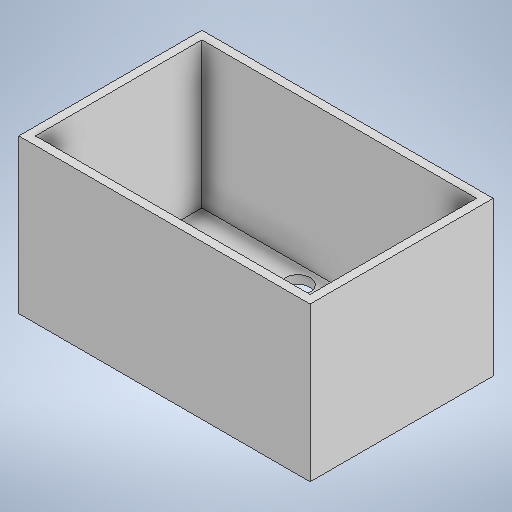
# Autodesk Inventor part: finalturnmotorcasing
Saved by Autodesk Inventor 2025.2 (Build 292293000, 293)
## iProperties
Created: 2026-03-25
Part Number: finalturnmotorcasing
Material: Generic
Document SubType Name: Modeling
Designer: hp
Density: 1 g/cm^3
Appearance: Default
Author: hp
Autodesk Inventor part; units mm, degrees
ref_plane "YZ Plane" through (0, 0, 0) normal (1, 0, 0) x (0, 1, 0)
ref_plane "XZ Plane" through (0, 0, 0) normal (0, 1, 0) x (-1, 0, 0)
ref_plane "XY Plane" through (0, 0, 0) normal (0, 0, 1) x (1, 0, 0)
sketch "Sketch1" plane through (0, 0, 0) normal (0, 1, 0) x (-1, 0, 0)
  line L0 (20.3745, 9.2758) -> (20.3745, -9.6242)
  line L1 (20.3745, 9.2758) -> (20.3745, -9.6242)
  circle A0 centre (24.4745, 4.8258) radius 2.25
  circle A1 centre (24.4745, 4.8258) radius 2.25
  line L2 (20.3745, 9.2758) -> (27.6745, 9.2758)
  line L3 (27.6745, 9.2758) -> (20.3745, 9.2758)
  line L4 (27.6745, 9.2758) -> (27.6745, -9.6242)
  line L5 (27.6745, 9.2758) -> (27.6745, -9.6242)
  circle A2 centre (24.4745, -5.1742) radius 2.25
  line L6 (20.3745, -9.6242) -> (27.6745, -9.6242)
  line L7 (27.6745, -9.6242) -> (20.3745, -9.6242)
  circle A3 centre (24.4745, -5.1742) radius 2.25
  line L8 (20.3745, 9.2758) -> (-20.1755, 9.2758)
  line L9 (20.3745, -9.6242) -> (-20.1755, -9.6242)
  line L10 (20.3745, 9.2758) -> (20.3745, -9.6242)
  line L11 (20.3745, 9.2758) -> (20.3745, -9.6242)
  line L12 (20.3745, 9.2758) -> (20.3745, -9.6242)
  line L13 (-20.1755, -9.6242) -> (20.3745, -9.6242)
  line L14 (-20.1755, -9.6242) -> (20.3745, -9.6242)
  line L15 (20.3745, 9.2758) -> (20.3745, -9.6242)
  line L16 (-20.1755, 9.2758) -> (20.3745, 9.2758)
  line L17 (-20.1755, 9.2758) -> (-20.1755, -9.6242)
  circle A4 centre (-10.3455, 0.2258) radius 6.5
  line L18 (20.3745, -9.6242) -> (-20.1755, -9.6242)
  line L19 (-20.1755, 9.2758) -> (-20.1755, -9.6242)
  line L20 (20.3745, 9.2758) -> (-20.1755, 9.2758)
  line L21 (20.3745, 9.2758) -> (20.3745, -9.6242)
  line L22 (20.3745, -9.6242) -> (-20.1755, -9.6242)
  line L23 (27.6745, -9.6242) -> (20.3745, -9.6242)
  line L24 (20.3745, -9.6242) -> (27.6745, -9.6242)
  line L25 (-20.1755, -9.6242) -> (20.3745, -9.6242)
  line L26 (-27.4755, -9.6242) -> (-20.1755, -9.6242)
  line L27 (-20.1755, -9.6242) -> (-27.4755, -9.6242)
  line L28 (-20.1755, 9.2758) -> (-27.4755, 9.2758)
  line L29 (-27.4755, 9.2758) -> (-20.1755, 9.2758)
  line L30 (-20.1755, 9.2758) -> (20.3745, 9.2758)
  line L31 (20.3745, 9.2758) -> (27.6745, 9.2758)
  line L32 (27.6745, 9.2758) -> (20.3745, 9.2758)
  line L33 (20.3745, 9.2758) -> (-20.1755, 9.2758)
  line L34 (-20.1755, 9.2758) -> (-20.1755, -9.6242)
  line L35 (-20.1755, 9.2758) -> (-20.1755, -9.6242)
  line L36 (-20.1755, 9.2758) -> (-20.1755, -9.6242)
  line L37 (-20.1755, 9.2758) -> (-20.1755, -9.6242)
  line L38 (-20.1755, 9.2758) -> (-20.1755, -9.6242)
  line L39 (-20.1755, 9.2758) -> (-20.1755, -9.6242)
  circle A5 centre (-24.3255, 4.8258) radius 2.25
  circle A6 centre (-24.3255, 4.8258) radius 2.25
  circle A7 centre (-24.3255, 4.8258) radius 2.25
  line L40 (-27.4755, 9.2758) -> (-20.1755, 9.2758)
  line L41 (-20.1755, -9.6242) -> (-27.4755, -9.6242)
  line L42 (-27.4755, 9.2758) -> (-27.4755, -9.6242)
  line L43 (-20.1755, 9.2758) -> (-27.4755, 9.2758)
  line L44 (-20.1755, 9.2758) -> (-20.1755, -9.6242)
  circle A8 centre (-24.3255, 4.8258) radius 2.25
  circle A9 centre (-24.3255, -5.1742) radius 2.25
  line L45 (-27.4755, -9.6242) -> (-20.1755, -9.6242)
  line L46 (-20.1755, 9.2758) -> (-20.1755, -9.6242)
  line L47 (-27.4755, 9.2758) -> (-20.1755, 9.2758)
  line L48 (-27.4755, 9.2758) -> (-27.4755, -9.6242)
  circle A10 centre (-24.3255, 4.8258) radius 2.25
  circle A11 centre (-24.3255, -5.1742) radius 2.25
  line L49 (-20.1755, 9.2758) -> (-20.1755, -9.6242)
  line L50 (-20.1755, 9.2758) -> (20.3745, 9.2758)
  circle A12 centre (-10.3455, 0.2258) radius 1.2002
  circle A13 centre (-10.3455, 0.2258) radius 2.9
  circle A14 centre (-10.3455, 0.2258) radius 6.5
  circle A15 centre (-10.3455, 0.2258) radius 6.5
  circle A16 centre (-10.3455, 0.2258) radius 6.5
  circle A17 centre (-10.3455, 0.2258) radius 6.5
  circle A18 centre (-10.3455, 0.2258) radius 2.9
  circle A19 centre (-10.3455, 0.2258) radius 6.5
  line L51 (-27.4755, 9.2758) -> (-27.4755, -9.6242)
  line L52 (-27.4755, 9.2758) -> (-27.4755, -9.6242)
  line L53 (-27.4755, 9.2758) -> (-27.4755, -9.6242)
  line L54 (-27.4755, 9.2758) -> (-27.4755, -9.6242)
  circle A20 centre (-24.3255, -5.1742) radius 2.25
  circle A21 centre (-24.3255, -5.1742) radius 2.25
  circle A22 centre (-24.3255, -5.1742) radius 2.25
  line L55 (-27.4755, -9.6242) -> (-20.1755, -9.6242)
  line L56 (-20.1755, -9.6242) -> (-27.4755, -9.6242)
  line L57 (20.3745, 9.2758) -> (20.3745, -9.6242)
  line L58 (20.3745, 9.2758) -> (20.3745, -9.6242)
  line L59 (20.3745, 9.2758) -> (20.3745, -9.6242)
  circle A23 centre (24.4745, 4.8258) radius 2.25
  circle A24 centre (24.4745, 4.8258) radius 2.25
  circle A25 centre (24.4745, -5.1742) radius 2.25
  circle A26 centre (24.4745, -5.1742) radius 2.25
  line L60 (27.6745, -9.6242) -> (20.3745, -9.6242)
  line L61 (20.3745, 9.2758) -> (20.3745, -9.6242)
  line L62 (27.6745, 9.2758) -> (20.3745, 9.2758)
  line L63 (27.6745, 9.2758) -> (27.6745, -9.6242)
  circle A27 centre (24.4745, 4.8258) radius 2.25
  circle A28 centre (24.4745, -5.1742) radius 2.25
  line L64 (20.3745, -9.6242) -> (27.6745, -9.6242)
  line L65 (27.6745, 9.2758) -> (27.6745, -9.6242)
  line L66 (20.3745, 9.2758) -> (27.6745, 9.2758)
  line L67 (20.3745, 9.2758) -> (20.3745, -9.6242)
  circle A29 centre (24.4745, 4.8258) radius 2.25
  circle A30 centre (24.4745, -5.1742) radius 2.25
  line L68 (27.6745, 9.2758) -> (27.6745, -9.6242)
  line L69 (27.6745, 9.2758) -> (27.6745, -9.6242)
  line L70 (-20.1755, 9.2758) -> (-20.1755, -9.6242)
  circle A31 centre (-10.3455, 0.2258) radius 1.2002
  circle A32 centre (-10.3455, 0.2258) radius 2.9
  circle A33 centre (-10.3455, 0.2258) radius 1.2002
  circle A34 centre (-10.3455, 0.2258) radius 2.9
  circle A35 centre (-10.3455, 0.2258) radius 1.2002
  circle A36 centre (-10.3455, 0.2258) radius 2.9
  circle A37 centre (-10.3455, 0.2258) radius 2.9
  circle A38 centre (-10.3455, 0.2258) radius 1.2002
  circle A39 centre (-10.3455, 0.2258) radius 1.2002
  circle A40 centre (-24.3255, 4.8258) radius 2.25
  circle A41 centre (-24.3255, -5.1742) radius 2.25
  line L71 (-20.1755, 9.2758) -> (-27.4755, 9.2758)
  line L72 (27.6745, -0.1742) -> (-27.4755, -0.1742)
  line L73 (0.0995, 9.2758) -> (0.0995, -9.6242)
  circle A42 centre (-10.3455, 0.2258) radius 20
  circle A43 centre (-10.3455, 0.2258) radius 22.5
  line L74 (-10.3455, 0.2258) -> (5.5644, -15.6841)
  line L75 (-10.3455, 0.2258) -> (12.1545, 0.2258) construction
  circle A44 centre (5.5644, -15.6841) radius 3
  circle A45 centre (5.5644, 16.1358) radius 3
  circle A46 centre (-26.2554, 16.1358) radius 3
  circle A47 centre (-26.2554, -15.6841) radius 3
  line L76 (35.0995, 21.8258) -> (-34.9005, 21.8258)
  line L77 (-34.9005, 21.8258) -> (-34.9005, -22.1742)
  line L78 (-34.9005, -22.1742) -> (35.0995, -22.1742)
  line L79 (35.0995, -22.1742) -> (35.0995, 21.8258)
  line L80 (35.0995, 21.8258) -> (-34.9005, -22.1742) construction
  line L81 (-34.9005, 21.8258) -> (35.0995, -22.1742) construction
  line L82 (33.0995, -20.1742) -> (-32.9005, -20.1742)
  line L83 (-32.9005, -20.1742) -> (-32.9005, 19.8258)
  line L84 (-32.9005, 19.8258) -> (33.0995, 19.8258)
  line L85 (33.0995, 19.8258) -> (33.0995, -20.1742)
  point P0 (0, 0)
  point P1 (0.0995, -0.1742)
  point P2 (-6.3655, 19.8258)
  point P3 (-14.3254, 19.8258)
  point P4 (-20.1755, -9.6242)
  dimension "d1" = 45
  dimension "d0" = 40
  dimension "d2" = 45
  dimension "d3" = 6
  dimension "d6" = 360
  dimension "d8" = 70
  dimension "d9" = 44
  dimension "d10" = 2
  constraints: 150 end point, 47 centre point, 7 midpoint, 4 parallel, 3 coincident, 2 horizontal, 2 perpendicular, 1 equal length, 48 other
  measures "d0" diameter of A42
  measures "d2" angle of L74 L75
  measures "d3" diameter of A44
  measures "d8" distance of L78.end L77.end
  measures "d9" distance of L77.end L76.end
  measures "d10" distance between parallel lines of L78 L82
extrude "Extrusion1" add sketch "Sketch1" against normal blind 2 contours L2 L4 L72 L0 | L8 A43 A45 L84 L85 L82 A44 L9 L6 L4 L2 | L0 L72 A43 L8 | L72 L4 L6 L0 | L0 L9 A43 L72 | A43 L72 A42 L8 | L8 A42 A45 A43 | A43 L9 A42 L72 | A42 L72 L73 L8 | L8 L28 L42 L26 L9 L74 A44 A42 A47 A46 L84 A45 | A43 A44 A42 L9 | A42 L9 L73 L72 | A45 A42 L84 A43 | A42 A44 L74 L9 | L17 L72 L42 L28 | L84 A42 A43 L76 | A43 L76 L79 L78 L82 L85 L84 | L17 L26 L42 L72 | L84 A42 | A43 L82 A47 A42 A44 | A42 A46 A43 L84 | A43 L84 L83 L82 L78 L77 L76 | A43 L78 L82 | A43 A46 A47 L82 L83 L84 | A42 A47 A43 A46
extrude "Extrusion2" add sketch "Sketch1" along normal blind 35 contours L84 A42 A43 L76 | A43 L76 L79 L78 L82 L85 L84 | L84 A42 | A43 L84 L83 L82 L78 L77 L76 | A43 L78 L82
body "Solid1"
